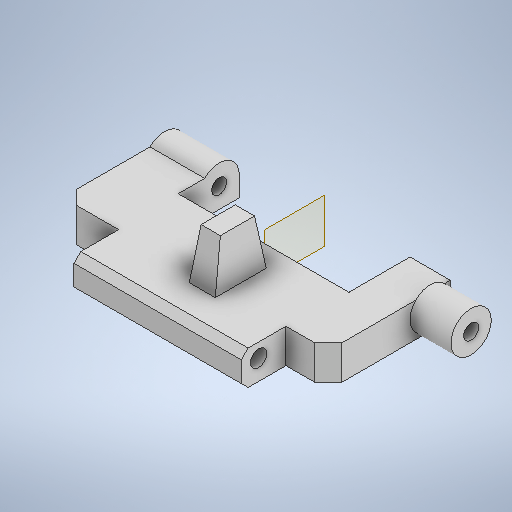
# Autodesk Inventor part: 履带片
Saved by Autodesk Inventor 2025.1 (Build 291241000, 241)
## iProperties
Created: 2025-08-28
Part Number: 履带片
Material: 常规
Document SubType Name: Modeling
Designer: Piw
Density: 1 g/cm^3
Appearance: 默认
Author: Piw
Autodesk Inventor part; units mm, degrees
ref_plane "YZ Plane" through (0, 0, 0) normal (1, 0, 0) x (0, 1, 0)
ref_plane "XZ Plane" through (0, 0, 0) normal (0, 1, 0) x (-1, 0, 0)
ref_plane "XY Plane" through (0, 0, 0) normal (0, 0, 1) x (1, 0, 0)
sketch "草图1" plane through (0, 0, 0) normal (1, 0, 0) x (0, 1, 0)
  circle A0 centre (4.0723, -9.46) radius 2.95
  line L0 (16.324, 0) -> (-17.1797, 0)
  line L1 (1.1223, -9.46) -> (1.1223, 0)
  line L2 (6.1223, 0) -> (6.1223, -7.3387)
  circle A1 centre (4.0723, 9.46) radius 1.2
  line L3 (6.1223, 0) -> (6.1223, 11)
  line L4 (1.1223, 0) -> (1.1223, 12)
  line L5 (1.1223, 12) -> (5.1223, 12)
  circle A2 centre (4.0723, -9.46) radius 1.1
  line L6 (5.1223, 12) -> (6.1223, 11)
  line L7 (4.0723, -12.41) -> (1.1223, -12.41)
  line L8 (1.1223, -12.41) -> (1.1223, -9.46)
  point P0 (0, 0)
  dimension "d0" = 5.9
  dimension "d2" = 18.92
  dimension "d3" = 2.4
  dimension "d4" = 5
  dimension "d5" = 2.2
  dimension "d8" = 135
  dimension "d9" = 24
  dimension "d10" = 1
  constraints: 18 end point, 4 vertical, 3 centre point, 3 perpendicular, 3 point on circle, 3 point on line, 2 coincident, 2 horizontal, 2 tangent, 1 symmetric about line
  measures "d0" diameter of A0
  measures "d2" diameter of A0.centre L0
  measures "d3" diameter of A1
  measures "d4" distance between parallel lines of L1 L2
  measures "d5" diameter of A2
  measures "d8" angle of L3 L6
  measures "d9" diameter of L5 L0
  measures "d10" horizontal distance of L5.end L3.end
extrude "拉伸1" add sketch "草图1" along normal blind 8
sketch "草图2" plane through (8, 0, 0) normal (1, 0, 0) x (0, 0, -1)
  line L0 (-11, 6.1223) -> (-12, 5.1223) projected
  line L1 (-12, 5.1223) -> (-12, 1.1223) projected
  line L2 (-12, 1.1223) -> (12.41, 1.1223) projected
  line L3 (12.41, 1.1223) -> (12.41, 4.0723) projected
  arc A0 (12.41, 4.0723) -> (7.3387, 6.1223) centre (9.46, 4.0723) ccw projected
  line L4 (7.3387, 6.1223) -> (-11, 6.1223) projected
  circle A1 centre (9.46, 4.0723) radius 1.1 projected
  circle A2 centre (-9.46, 4.0723) radius 1.2 projected
  line L5 (7.3387, 6.1223) -> (-11, 6.1223) projected
  line L6 (5.46, 6.1223) -> (5.46, 1.1223)
  point P0 (0, 0)
  point P1 (5.46, 3.6223)
  dimension "d11" = 4
  constraints: 2 end point, 2 point on line, 1 midpoint, 1 perpendicular
  measures "d11" horizontal distance of A0.centre point (5.46, 3.622)
extrude "拉伸2" add sketch "草图2" along normal blind 25 contours L4 L6 L2 L1 L0
sketch "草图3" plane through (33, 0, 0) normal (1, 0, 0) x (0, 0, -1)
  line L0 (-12, 1.1223) -> (5.46, 1.1223) projected
  line L1 (5.46, 1.1223) -> (5.46, 6.1223) projected
  line L2 (5.46, 6.1223) -> (-11, 6.1223) projected
  line L3 (-11, 6.1223) -> (-12, 5.1223) projected
  line L4 (-12, 5.1223) -> (-12, 1.1223) projected
  circle A0 centre (-9.46, 4.0723) radius 1.2 projected
  line L5 (-12, 1.1223) -> (12.41, 1.1223) projected
  line L6 (5.46, 1.1223) -> (12.41, 1.1223)
  line L7 (12.41, 1.1223) -> (12.41, 6.1223)
  line L8 (12.41, 6.1223) -> (5.46, 6.1223)
  circle A1 centre (9.46, 4.0723) radius 1.1 projected
  arc A2 (12.41, 4.0723) -> (7.3387, 6.1223) centre (9.46, 4.0723) ccw projected
  point P0 (0, 0)
  constraints: 6 end point, 2 perpendicular, 1 collinear, 1 tangent
extrude "拉伸3" add sketch "草图3" along normal blind 5.9 contours L4 L3 L2 L1 L0 | L1 L8 A2 L7 L5 | A2 L8 L7
sketch "草图4" plane through (38.9, 0, 0) normal (1, 0, 0) x (0, 0, -1)
  circle A0 centre (9.46, 4.0723) radius 1.1 projected
  circle A1 centre (9.46, 4.0723) radius 2.95
  line L0 (-12, 1.1223) -> (12.41, 1.1223) projected
  point P0 (0, 0)
  point P1 (8.9146, 1.1223)
  point P2 (9.46, 1.1223)
  dimension "d16" = 5.9
  constraints: 1 centre point, 1 coincident
  measures "d16" diameter of A1
extrude "拉伸4" add sketch "草图4" along normal blind 6
chamfer "倒角1" distance 2 angle 45 1 edges at (20.5, 6.1223, -5.46)
chamfer "倒角2" distance 1 angle 45 1 edges at (19.45, 1.1223, 12)
chamfer "倒角3" distance 1 angle 45 1 edges at (20.5, 1.1223, -5.46)
sketch "草图5" plane through (0, 0, 0) normal (-1, 0, 0) x (0, 0, 1)
  line L0 (-7.3387, 6.1223) -> (11, 6.1223) projected
  line L1 (5.46, 6.1223) -> (5.46, 1.1223)
  line L2 (11, 1.1223) -> (-12.41, 1.1223) projected
  circle A0 centre (9.46, 4.0723) radius 1.2 projected
  line L3 (12, 5.1223) -> (12, 2.1223) projected
  line L4 (11, 6.1223) -> (12, 5.1223) projected
  line L5 (12, 2.1223) -> (11, 1.1223) projected
  point P0 (0, 0)
  dimension "d28" = 4
  constraints: 2 end point, 2 point on line, 1 vertical
  measures "d28" distance from line of L1 A0.centre
extrude "拉伸5" cut sketch "草图5" against normal blind 8.2
sketch "草图6" plane through (38.9, 0, 0) normal (1, 0, 0) x (0, 0, -1)
  line L0 (-12, 5.1223) -> (-12, 2.1223) projected
  line L1 (-11, 6.1223) -> (-12, 5.1223) projected
  line L2 (-5.46, 6.1223) -> (-11, 6.1223) projected
  line L3 (-5.46, 1.1223) -> (-5.46, 6.1223) projected
  line L4 (-11, 1.1223) -> (-5.46, 1.1223) projected
  line L5 (-12, 2.1223) -> (-11, 1.1223) projected
  circle A0 centre (-9.46, 4.0723) radius 1.2 projected
  point P0 (0, 0)
extrude "拉伸6" cut sketch "草图6" against normal blind 6.2
chamfer "倒角5" distance 2 angle 45 2 edges at (38.9, 3.6223, 5.46) (0, 3.6223, 5.46)
ref_plane "工作平面1" through (20.1, 0, 0) normal (1, 0, 0) x (0, 0, -1)
sketch "草图7" plane through (20.1, 0, 0) normal (1, 0, 0) x (0, 0, -1)
  line L0 (7.3387, 6.1223) -> (-3.46, 6.1223) projected
  line L1 (0.46, 6.1223) -> (-0.7743, 13.1223)
  line L2 (-0.7743, 13.1223) -> (-5.7743, 13.1223)
  line L3 (-5.7743, 13.1223) -> (-7.0086, 6.1223)
  line L4 (-7.0086, 6.1223) -> (0.46, 6.1223)
  point P0 (0, 0)
  point P1 (7.2697, 6.1223)
  point P2 (3.46, 6.1223)
  point P3 (-3.46, 6.1223)
  dimension "d40" = 80
  dimension "d41" = 80
  dimension "d42" = 5
  dimension "d43" = 3
  dimension "d44" = 7
  constraints: 8 end point, 1 collinear, 1 horizontal, 1 point on line
  measures "d40" angle of L0 L1
  measures "d41" angle of L4 L3
  measures "d42" distance of L1.end L2.end
  measures "d43" distance of point (3.46, 6.122) L1.start
  measures "d44" distance between parallel lines of L0 L2
extrude "拉伸7" add sketch "草图7" along normal blind 3.8
sketch "草图8" plane through (8.2, 2.1223, 12) normal (0, 0, 1) x (1, 0, 0)
  line L0 (11.9, 11) -> (15.7, 11) projected
  line L1 (11.9, 11) -> (11.9, 4) projected
  line L2 (12.3895, 11) -> (11.9, 4)
  line L3 (15.7, 11) -> (15.7, 4) projected
  line L4 (15.2105, 11) -> (15.7, 4)
  line L5 (11.9, 4) -> (15.7, 4) projected
  line L6 (15.7, 4) -> (11.9, 4)
  point P0 (-8.2, -2.1223)
  dimension "d47" = 86
  dimension "d48" = 86
  constraints: 6 end point, 2 point on line, 1 collinear
  measures "d47" angle of L5 L4
  measures "d48" angle of L5 L2
extrude "拉伸8" cut sketch "草图8" against normal blind 100 contours L0 L2 L1 | L0 L3 L4
